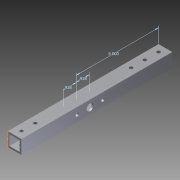
# Autodesk Inventor part: shooter 9 inch horizontal
Saved by Autodesk Inventor 2011 SP1 (Build 150282100, 282)
## iProperties
Created: 2012-01-18
Part Number: shooter 9 inch horizontal
Document SubType Name: Modeling
Designer: Christopher
Density: 1 g/cm^3
Author: Christopher
Autodesk Inventor part; units mm, degrees
ref_plane "YZ Plane" through (0, 0, 0) normal (1, 0, 0) x (0, 1, 0)
ref_plane "XZ Plane" through (0, 0, 0) normal (0, 1, 0) x (-1, 0, 0)
ref_plane "XY Plane" through (0, 0, 0) normal (0, 0, 1) x (1, 0, 0)
sketch "Sketch1" plane through (0, 0, 0) normal (0, 0, 1) x (1, 0, 0)
  line L0 (0, 0) -> (25.4, 0)
  line L1 (25.4, 0) -> (25.4, 25.4)
  line L2 (25.4, 25.4) -> (0, 25.4)
  line L3 (0, 25.4) -> (0, 0)
  line L4 (3.175, 22.225) -> (22.225, 22.225)
  line L5 (22.225, 22.225) -> (22.225, 3.175)
  line L6 (22.225, 3.175) -> (3.175, 3.175)
  line L7 (3.175, 3.175) -> (3.175, 22.225)
  dimension "d0" = 25.4
  dimension "d1" = 25.4
  dimension "d2" = 3.175
  constraints: 16 end point, 4 parallel, 2 perpendicular, 1 horizontal, 3 other
  measures "d0" distance of L1.end L2.end
  measures "d1" distance of L0.end L1.end
  measures "d2" distance between parallel lines of L3 L7
extrude "Extrusion1" add sketch "Sketch1" against normal blind 279.4
sketch "Sketch2" plane through (0, 25.4, 0) normal (0, 1, 0) x (1, 0, 0)
  line L0 (25.4, 279.4) -> (0, 279.4) projected
  line L1 (25.4, 0) -> (0, 0) projected
  point P0 (12.7, 266.7)
  point P1 (12.7, 241.3)
  point P2 (12.7, 215.9)
  point P3 (12.7, 12.7)
  point P4 (12.7, 38.1)
  dimension "d5" = 25.4
  dimension "d6" = 12.7
  dimension "d7" = 25.4
  dimension "d8" = 25.4
  dimension "d9" = 12.7
  measures "d5" distance of point (12.7, 38.1) point (12.7, 12.7)
  measures "d6" distance from line of L1 point (12.7, 12.7)
  measures "d7" distance of point (12.7, 241.3) point (12.7, 215.9)
  measures "d8" distance of point (12.7, 241.3) point (12.7, 266.7)
  measures "d9" distance from line of L0 point (12.7, 266.7)
hole "Hole1" at (12.7, 25.4, -266.7) at (12.7, 25.4, -241.3) at (12.7, 25.4, -215.9) at (12.7, 25.4, -12.7) at (12.7, 25.4, -38.1) direction (0, -1, 0) diameter 6.35 depth 25.4 tip angle 118
sketch "Sketch3" plane through (0, 0, 0) normal (-1, 0, 0) x (0, 0, 1)
  line L0 (-279.4, 25.4) -> (-279.4, 0) projected
  line L1 (0, 25.4) -> (0, 0) projected
  point P0 (-127, 12.7)
  point P1 (-103.1875, 12.7)
  point P2 (-150.8125, 12.7)
  point P3 (0, 12.7)
  dimension "d17" = 152.4
  dimension "d18" = 23.8125
  dimension "d19" = 23.8125
  constraints: 3 horizontal alignment, 1 midpoint
  measures "d17" distance from line of L0 point (-127, 12.7)
  measures "d18" distance of point (-150.812, 12.7) point (-127, 12.7)
  measures "d19" distance of point (-127, 12.7) point (-103.188, 12.7)
hole "Hole2" at (0, 12.7, -103.1875) at (0, 12.7, -150.8125) direction (1, 0, 0) diameter 6.35 depth 25.4 tip angle 118
hole "Hole3" at (0, 12.7, -127) direction (1, 0, 0) diameter 12.7 depth 25.4 tip angle 118
body "Solid1"
